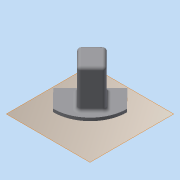
# Autodesk Inventor part: palette_push
Saved by Autodesk Inventor 2017 (Build 210142000, 142)
## iProperties
Created: 2018-05-06
Part Number: palette_push
Material: Generic
Document SubType Name: Modeling
Designer: Aegir
Density: 1 g/cm^3
Appearance: Default
Author: Aegir
Autodesk Inventor part; units mm, degrees
ref_plane "YZ Plane" through (0, 0, 0) normal (1, 0, 0) x (0, 1, 0)
ref_plane "XZ Plane" through (0, 0, 0) normal (0, 1, 0) x (-1, 0, 0)
ref_plane "XY Plane" through (0, 0, 0) normal (0, 0, 1) x (1, 0, 0)
ref_plane "Plan de construction1" through (0, 0, 0) normal (0, 0, 1) x (1, 0, 0)
sketch "Esquisse1" plane through (0, 0, 0) normal (0, 0, 1) x (1, 0, 0)
  line L0 (12.600402, 13.369459) -> (-37.128252, -35.732002)
  line L1 (-42.505343, -6.84222) -> (-16.505712, -33.167478)
  line L2 (8.432313, -8.537922) -> (-17.567318, 17.787336)
  line L3 (-17.567318, 17.787336) -> (-42.505343, -6.84222)
  spline S0 degree 3 poles (-30.559567, -18.937609) (-29.251135, -19.178539) (-27.810091, -19.446017) (-24.924717, -19.685136) (-23.47934, -19.643963) (-21.695605, -19.298823) (-21.177712, -19.167045) (-20.168818, -18.825553) (-19.677941, -18.615468) (-18.84768, -18.187738) (-18.426343, -17.934552) (-17.631099, -17.362687) (-17.257309, -17.043846) (-16.938864, -16.72934) knots 0 0 0 0 0.39912855 0.39912855 0.7982571 0.7982571 0.94417416 0.94417416 1.09009122 1.09009122 1.22436299 1.22436299 1.35863477 1.35863477 1.35863477 1.35863477
  spline S1 degree 3 poles (-7.999161, -7.900216) (-7.680716, -7.58571) (-7.357248, -7.215917) (-6.77553, -6.427852) (-6.517119, -6.009699) (-6.079089, -5.184826) (-5.862912, -4.696602) (-5.508889, -3.692036) (-5.370676, -3.175823) (-5.003363, -1.396522) (-4.944203, 0.048231) (-5.147393, 2.936358) (-5.396916, 4.380619) (-5.621542, 5.691948) knots 3.77145385 3.77145385 3.77145385 3.77145385 3.90572563 3.90572563 4.0399974 4.0399974 4.18591446 4.18591446 4.33183152 4.33183152 4.73096007 4.73096007 5.13008862 5.13008862 5.13008862 5.13008862
  line L4 (-16.938864, -16.72934) -> (-7.999161, -7.900216)
  line L5 (-17.567318, 17.787336) -> (-5.621542, 5.691948)
  line L6 (-17.567318, 17.787336) -> (-42.505343, -6.84222)
  line L7 (-42.505343, -6.84222) -> (-30.559567, -18.937609)
  arc A0 (-30.559567, -18.937609) -> (-5.621542, 5.691948) centre (-30.176225, 5.614205) ccw
  point P0 (0, 0)
extrude "Extrusion1" add sketch "Esquisse1" along normal blind 2 contours A0 L0 L1 L3 L2 | A0 L0
sketch "Esquisse2" plane through (0, 0, 2) normal (0, 0, 1) x (1, 0, 0)
  line L0 (37.657428, -63.069018) -> (-69.549529, 45.480633)
  line L1 (37.657428, -63.069018) -> (-69.549529, 45.480633)
  line L2 (-29.434692, -3.955721) -> (-33.278207, -0.064069)
  line L3 (-33.278207, -0.064069) -> (-23.285586, 9.804949)
  line L4 (-23.285586, 9.804949) -> (-19.442072, 5.913297)
  line L5 (-24.775557, -8.673208) -> (-20.790583, -12.708092)
  line L6 (-20.790583, -12.708092) -> (-10.797962, -2.839074)
  line L7 (-10.797962, -2.839074) -> (-14.782937, 1.195809)
  line L8 (-24.775557, -8.673208) -> (-29.434692, -3.955721)
  line L9 (-19.442072, 5.913297) -> (-14.782937, 1.195809)
  point P0 (0, 0)
  point P1 (-20.366346, -4.318536)
  constraints: 20 end point, 1 parallel, 1 perpendicular, 1 point on line, 6 other
extrude "Extrusion2" add sketch "Esquisse2" along normal blind 10
sketch "Esquisse6" plane through (-23.285586, 9.804949, 12) normal (0.7114935, 0.7026927, 0) x (0, 0, -1)
  line L0 (0, 0) -> (-15.824808, 0)
  line L1 (-15.824808, 0) -> (-15.824808, -17.771102)
  line L2 (-15.824808, -17.771102) -> (0, -17.771102)
  line L3 (0, -17.771102) -> (0, 0)
  point P0 (12, -23.338769)
  point P1 (0, -17.771102)
  constraints: 8 end point, 2 parallel, 1 coincident, 1 horizontal, 1 perpendicular
extrude "Extrusion6" add sketch "Esquisse6" against normal up to surface (14.044571 mm away)
fillet "Congé4" radius 2 8 edges at (-33.2782, -0.0641, 14.9124) (-23.2856, 9.8049, 14.9124) (-20.7906, -12.7081, 14.9124) (-15.7943, -7.7736, 2) (-17.0418, 3.4829, 2) (-27.0344, -6.3861, 2) (-28.2819, 4.8704, 2) (-10.798, -2.8391, 14.9124)
fillet_without_effect "Congé6"
fillet "Congé7" radius 2 8 edges at (-11.6264, -2.8339, 27.8248) (-32.4498, -0.0692, 27.8248) (-20.7854, -11.8797, 27.8248) (-15.7943, -7.7736, 27.8248) (-23.2907, 8.9765, 27.8248) (-17.0418, 3.4829, 27.8248) (-28.2819, 4.8704, 27.8248) (-27.0344, -6.3861, 27.8248)
